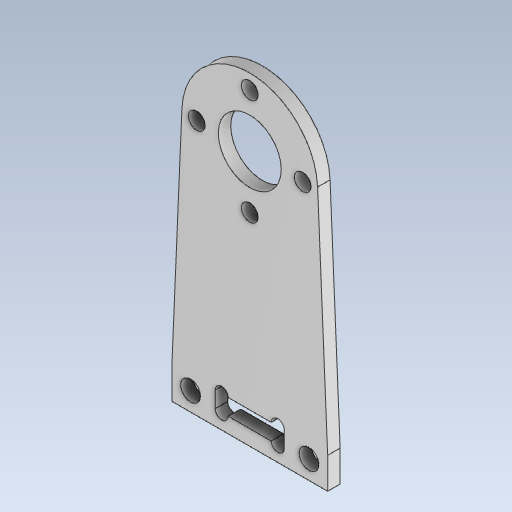
# Autodesk Inventor part: Foot_back_frame
Saved by Autodesk Inventor 2020.4 (Build 244396000, 396)
## iProperties
Part Number: Foot_back_frame
Material: アルミニウム 2014-T4
Document SubType Name: Modeling
Designer: Masato Kubotera
Density: 2.8 g/cm^3
Appearance: 滑らか - 淡い灰色
Description: A2017 T2
Mass: 5.59731 g
Surface Area: 25.1759 cm^2
Volume: 1.99904 cm^3
Author: Masato Kubotera
Autodesk Inventor part; units mm, degrees
ref_plane "YZ Plane" through (0, 0, 0) normal (1, 0, 0) x (0, 1, 0)
ref_plane "XZ Plane" through (0, 0, 0) normal (0, 1, 0) x (-1, 0, 0)
ref_plane "XY Plane" through (0, 0, 0) normal (0, 0, 1) x (1, 0, 0)
sketch "スケッチ1" plane through (0, 0, 0) normal (1, 0, 0) x (0, 1, 0)
  circle A0 centre (0, 0) radius 5.05
  line L0 (-10.9106, 0) -> (10.9106, 0) construction
  line L1 (0, 11.25) -> (0, -41) construction
  line L2 (-10.8894, 0.4808) -> (-12.5, -36)
  line L3 (-12.5, -36) -> (-12.5, -41)
  line L4 (-12.5, -41) -> (12.5, -41)
  circle A1 centre (0, 8.5) radius 1.35
  circle A2 centre (0, 8.5) radius 2.4 construction
  circle A3 centre (-8.5, 0) radius 1.35
  circle A4 centre (0, -8.5) radius 1.35
  circle A5 centre (8.5, 0) radius 1.35
  line L5 (5.5, -36) -> (-5.5, -36) construction
  line L6 (-5.5, -36) -> (-5.5, -38.5) construction
  line L7 (-5.5, -38.5) -> (5.5, -38.5) construction
  line L8 (5.5, -38.5) -> (5.5, -36) construction
  line L9 (5.5, -36) -> (-5.5, -38.5) construction
  line L10 (-5.5, -36) -> (5.5, -38.5) construction
  circle A6 centre (-9.5, -38) radius 1.6
  line L11 (-12.5, -38) -> (12.1081, -38) construction
  circle A7 centre (-9.5, -38) radius 2.75 construction
  line L12 (-5.55, -35.95) -> (5.55, -35.95)
  line L13 (5.55, -35.95) -> (5.55, -38.55)
  line L14 (5.55, -38.55) -> (-5.55, -38.55)
  line L15 (-5.55, -38.55) -> (-5.55, -35.95)
  line L16 (-5.55, -35.95) -> (5.55, -38.55) construction
  line L17 (5.55, -35.95) -> (-5.55, -38.55) construction
  arc A8 (-3.45, -35.95) -> (-5.55, -35.95) centre (-4.5, -35.95) ccw
  line L18 (-5.5, -37.25) -> (5.5, -37.25) construction
  arc A9 (-5.55, -38.55) -> (-3.45, -38.55) centre (-4.5, -38.55) ccw
  line L19 (10.8894, 0.4808) -> (12.5, -36)
  line L20 (12.5, -36) -> (12.5, -41)
  circle A10 centre (9.5, -38) radius 1.6
  circle A11 centre (9.5, -38) radius 2.75 construction
  arc A12 (5.55, -35.95) -> (3.45, -35.95) centre (4.5, -35.95) ccw
  arc A13 (3.45, -38.55) -> (5.55, -38.55) centre (4.5, -38.55) ccw
  arc A14 (10.8894, 0.4808) -> (-10.8894, 0.4808) centre (0, 0) ccw
  line L21 (-13.5, 1) -> (13.5, 1) construction
  circle A15 centre (-13.5, 1) radius 2.4 construction
  point P0 (0, -37.25)
  point P1 (3.45, -35.95)
  point P2 (0, 1)
  dimension "d0" = 10.1
  dimension "d1" = 5
  dimension "d2" = 41
  dimension "d3" = 25
  dimension "d4" = 2.7
  dimension "d5" = 8.5
  dimension "d6" = 4.8
  dimension "d9" = 360
  dimension "d11" = 11
  dimension "d12" = 2.5
  dimension "d13" = 3.2
  dimension "d14" = 5.5
  dimension "d15" = 3
  dimension "d16" = 0.05
  dimension "d17" = 0.05
  dimension "d18" = 1.05
  dimension "d19" = 19
  dimension "d22" = 27
  dimension "d23" = 1
  dimension "d25" = 4.8
  constraints: 44 end point, 16 centre point, 11 point on line, 10 midpoint, 10 point on circle, 10 symmetric about line, 6 coincident, 5 horizontal, 4 parallel, 4 perpendicular, 2 tangent, 1 vertical, 14 other
  measures "d0" diameter of A0
  measures "d1" distance of L2.end L3.end
  measures "d2" vertical distance of L3.end point (0, 0)
  measures "d3" distance of L3.end L4.end
  measures "d4" diameter of A1
  measures "d5" distance of point (0, 0) A1.centre
  measures "d6" diameter of A2
  measures "d11" distance of L7.end L6.end
  measures "d12" distance of L6.end L5.end
  measures "d13" diameter of A6
  measures "d14" diameter of A7
  measures "d15" distance of L3.end L11.start
  measures "d16" distance from line of L12.start L5
  measures "d17" distance between parallel lines of L15 L6
  measures "d18" radius of A8
  measures "d19" distance of A11.centre A6.centre
  measures "d22" distance of L21.start L21.end
  measures "d23" distance of point (0, 0) point (0, 1)
  measures "d25" diameter of A15
extrude "押し出し1" add sketch "スケッチ1" along normal blind 2
equation "\"d17\" = d16"
